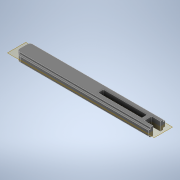
# Autodesk Inventor part: GT2RackA
Saved by Autodesk Inventor 2022 (Build 260153000, 153)
## iProperties
Created: 2022-08-08
Part Number: GT2RackA
Material: UHMW, negro
Document SubType Name: Modeling
Designer: JK
Density: 0.94 g/cm^3
Appearance: Suave - Negro
Author: JK
Autodesk Inventor part; units mm, degrees
ref_plane "YZ Plane" through (0, 0, 0) normal (1, 0, 0) x (0, 1, 0)
ref_plane "XZ Plane" through (0, 0, 0) normal (0, 1, 0) x (-1, 0, 0)
ref_plane "XY Plane" through (0, 0, 0) normal (0, 0, 1) x (1, 0, 0)
sketch "Boceto1" plane through (0, 0, 0) normal (0, 1, 0) x (-1, 0, 0)
  line L0 (96, 7.5) -> (-96, 7.5)
  line L1 (-96, 7.5) -> (-96, -7.5)
  line L2 (-96, -7.5) -> (96, -7.5)
  line L3 (96, -7.5) -> (96, 7.5)
  line L4 (96, 7.5) -> (-96, -7.5) construction
  line L5 (-96, 7.5) -> (96, -7.5) construction
  point P0 (0, 0)
  dimension "d0" = 192
  dimension "d1" = 15
  constraints: 12 end point, 2 midpoint, 2 parallel, 1 horizontal, 1 perpendicular
  measures "d0" distance between parallel lines of L3 L1
  measures "d1" distance of L2.end L0.start
extrude "Extrusión1" add sketch "Boceto1" along normal blind 10
sketch "Boceto2" plane through (0, 0, 0) normal (1, 0, 0) x (0, 1, 0)
  line L0 (0, 7.5) -> (10, 7.5) projected
  line L1 (2.1, 7.5) -> (7.9, 7.5)
  line L2 (7.9, 7.5) -> (7.9, 9.5)
  line L3 (7.9, 9.5) -> (2.1, 9.5)
  line L4 (2.1, 9.5) -> (2.1, 7.5)
  line L5 (0, -7.5) -> (0, 7.5) projected
  line L6 (0, -7.5) -> (10, -7.5) projected
  line L7 (2.1, -7.5) -> (7.9, -7.5)
  line L8 (7.9, -7.5) -> (7.9, -9.5)
  line L9 (7.9, -9.5) -> (2.1, -9.5)
  line L10 (2.1, -9.5) -> (2.1, -7.5)
  point P0 (0, 0)
  point P1 (7.9, -7.5)
  dimension "d4" = 5.8
  dimension "d5" = 2.1
  dimension "d6" = 2
  constraints: 16 end point, 4 parallel, 3 collinear, 2 horizontal, 2 perpendicular, 2 point on line
  measures "d4" distance between parallel lines of L4 L2
  measures "d5" distance between parallel lines of L5 L4
  measures "d6" distance between parallel lines of L0 L3
extrude "Extrusión2" add sketch "Boceto2" along normal mid plane 192
sketch "Boceto4" plane through (-96, 0, -7.5) normal (-1, 0, 0) x (0, 0, 1)
  line L0 (15, 2.1) -> (17, 2.1) projected
  line L1 (0, 7.9) -> (-2, 7.9) projected
  line L2 (17, 2.1) -> (-2, 2.1)
  line L3 (-2, 2.1) -> (-2, 7.9)
  line L4 (-2, 7.9) -> (17, 7.9)
  line L5 (17, 7.9) -> (17, 2.1)
  point P0 (7.5, 0)
  constraints: 8 end point, 2 parallel, 1 horizontal, 1 perpendicular
extrude "Extrusión3" cut sketch "Boceto4" against normal blind 1
sketch "Boceto5" plane through (96, 0, 7.5) normal (1, 0, 0) x (0, 0, -1)
  line L0 (0, 7.9) -> (-2, 7.9) projected
  line L1 (17, 2.1) -> (17, 7.9) projected
  line L2 (-2, 7.9) -> (17, 7.9)
  line L3 (17, 7.9) -> (17, 2.1)
  line L4 (17, 2.1) -> (-2, 2.1)
  line L5 (-2, 2.1) -> (-2, 7.9)
  point P0 (7.5, 0)
  constraints: 8 end point, 2 parallel, 1 horizontal, 1 perpendicular
extrude "Extrusión4" cut sketch "Boceto5" against normal blind 1
fillet "Empalme1" radius 5 4 edges at (95, 5, -9.5) (95, 5, 9.5) (-95, 5, -9.5) (-95, 5, 9.5)
fillet "Empalme2" radius 3 8 edges at (96, 8.95, 7.5) (96, 1.05, 7.5) (96, 8.95, -7.5) (96, 1.05, -7.5) (-96, 1.05, 7.5) (-96, 8.95, 7.5) (-96, 1.05, -7.5) (-96, 8.95, -7.5)
sketch "Boceto7" plane through (0, 10, 0) normal (0, 1, 0) x (1, 0, 0)
  line L0 (-90, 9.5) -> (90, 9.5) projected
  line L1 (-90, -9.5) -> (90, -9.5) projected
  line L2 (82.6935, 4) -> (-107.9962, 4)
  line L3 (-107.9962, 4) -> (-107.9962, -4)
  line L4 (-107.9962, -4) -> (82.6935, -4)
  line L5 (82.6935, -4) -> (82.6935, 4)
  line L6 (93, 7.5) -> (-93, 7.5) projected
  line L7 (96, 9.5) -> (66, 9.5)
  line L8 (66, 9.5) -> (66, -22.8831)
  line L9 (66, -22.8831) -> (96, -22.8831)
  line L10 (96, -22.8831) -> (96, 9.5)
  line L11 (96, -4.5) -> (96, 4.5) projected
  line L12 (66, 9.5) -> (56, 9.5)
  line L13 (56, 9.5) -> (56, 4)
  line L14 (56, 4) -> (66, 4)
  line L15 (66, 4) -> (66, 9.5)
  line L16 (66, -9.5) -> (56, -9.5)
  line L17 (56, -9.5) -> (56, -4)
  line L18 (56, -4) -> (66, -4)
  line L19 (66, -4) -> (66, -9.5)
  line L20 (66, 4) -> (46, 4)
  line L21 (46, 4) -> (46, -4)
  line L22 (46, -4) -> (66, -4)
  line L23 (66, -4) -> (66, 4)
  point P0 (90, 9.5)
  point P1 (66, 4)
  point P2 (66, -4)
  dimension "d17" = 8
  dimension "d18" = 3.5
  dimension "d19" = 30
  dimension "d20" = 10
  dimension "d23" = 10
  constraints: 40 end point, 10 parallel, 5 horizontal, 5 perpendicular, 5 point on line, 4 collinear
  measures "d17" distance of L4.end L2.start
  measures "d18" distance between parallel lines of L6 L2
  measures "d19" distance between parallel lines of L10 L8
  measures "d20" distance between parallel lines of L15 L13
  measures "d23" distance between parallel lines of L13 L21
extrude "Extrusión5" cut sketch "Boceto7" against normal through all contours L0 L8 L6 L13 | L0 L7 L10 L9 L8 L4 L5 L2 | L6 L8 L2 L13 | L2 L8 L4 L21 | L2 L5 L4 L8 | L8 L1 L17 L4
sketch "Boceto8" plane through (0, 10, 0) normal (0, 1, 0) x (1, 0, 0)
  line L0 (56, -0.8) -> (56, -7.5)
  line L1 (46, 4.15) -> (56, 4.15)
  line L2 (56, 4.15) -> (56, -4.15)
  line L3 (56, -4.15) -> (46, -4.15)
  line L4 (46, -4.15) -> (46, 4.15)
  line L5 (46, -4) -> (46, 4) projected
  line L6 (46, 4) -> (56, 4) projected
  line L7 (56, -4) -> (46, -4) projected
  point P0 (0, 0)
  dimension "d24" = 0.15
  dimension "d25" = 0.15
  constraints: 10 end point, 2 parallel, 1 collinear, 1 horizontal, 1 midpoint, 1 perpendicular
  measures "d24" distance between parallel lines of L1 L6
  measures "d25" distance between parallel lines of L7 L3
extrude "Extrusión6" cut sketch "Boceto8" against normal through all
sketch "Boceto10" plane through (46, 10, 4.15) normal (1, 0, 0) x (0, 0, -1)
  circle A0 centre (4.15, -5) radius 1.7
  line L0 (8.3, -10) -> (0, -10) projected
  point P0 (4.15, -10)
  point P1 (4.15, -10)
  dimension "d35" = 3.4
  dimension "d36" = 5
  constraints: 1 centre point, 1 midpoint, 1 vertical alignment
  measures "d35" diameter of A0
  measures "d36" distance from line of A0.centre L0
extrude "Extrusión8" cut sketch "Boceto10" against normal blind 7.5
sketch "Boceto11" plane through (0, 10, 0) normal (0, 1, 0) x (1, 0, 0)
  line L0 (-8, -2.8775) -> (42, -2.8775)
  line L1 (42, -2.8775) -> (42, 3.1225)
  line L2 (42, 3.1225) -> (-8, 3.1225)
  line L3 (-8, 3.1225) -> (-8, -2.8775)
  line L4 (46, -4.15) -> (46, 4.15) projected
  point P0 (0, 0)
  dimension "d39" = 6
  dimension "d40" = 50
  dimension "d41" = 4
  constraints: 8 end point, 2 parallel, 1 horizontal, 1 perpendicular
  measures "d39" distance between parallel lines of L2 L0
  measures "d40" distance of L0.start L0.end
  measures "d41" distance between parallel lines of L1 L4
extrude "Extrusión9" cut sketch "Boceto11" against normal through all
ref_plane "Plano de trabajo1" through (-95, 5, 4.5) normal (0, 1, 0) x (1, 0, 0)
sketch "Boceto12" plane through (-95, 5, 4.5) normal (0, 1, 0) x (1, 0, 0)
  arc A0 (0.8333, 11.7639) -> (-1, 9) centre (2, 9) ccw projected
  arc A1 (0.8333, 11.7639) -> (0, 9) centre (5, 9) ccw projected
  line L0 (0, 9) -> (0, 0) projected
  arc A2 (0, 0) -> (0.8333, -2.7639) centre (5, 0) ccw projected
  arc A3 (-1, 0) -> (0.8333, -2.7639) centre (2, 0) ccw projected
  line L1 (-1, 9) -> (-1, 0) projected
  point P0 (95, 4.5)
extrude "Extrusión10" cut sketch "Boceto12" along normal mid plane 6.6
sketch "Boceto9" plane through (0, 10, 0) normal (0, 1, 0) x (1, 0, 0)
  line L0 (38.5, 3) -> (42, 3)
  line L1 (42, 3) -> (42, -3)
  line L2 (42, -3) -> (38.5, -3)
  line L3 (38.5, -3) -> (38.5, 3)
  line L4 (38.5, 3) -> (42, -3) construction
  line L5 (42, 3) -> (38.5, -3) construction
  line L6 (46, -4.15) -> (46, 4.15) projected
  line L7 (42, 1.75) -> (46, 1.75)
  line L8 (46, 1.75) -> (46, -1.75)
  line L9 (46, -1.75) -> (42, -1.75)
  line L10 (42, -1.75) -> (42, 1.75)
  point P0 (0, 0)
  point P1 (40.25, 0)
  dimension "d28" = 6
  dimension "d29" = 3.5
  dimension "d30" = 1.75
  dimension "d31" = 3.5
  dimension "d32" = 4
  constraints: 20 end point, 4 parallel, 2 horizontal, 2 midpoint, 2 perpendicular, 2 point on line
  measures "d28" distance of L2.end L0.start
  measures "d29" distance of L0.start L0.end
  measures "d30" distance from line of L7 point (40.25, 0)
  measures "d31" distance between parallel lines of L9 L7
  measures "d32" distance of L7.start L7.end
